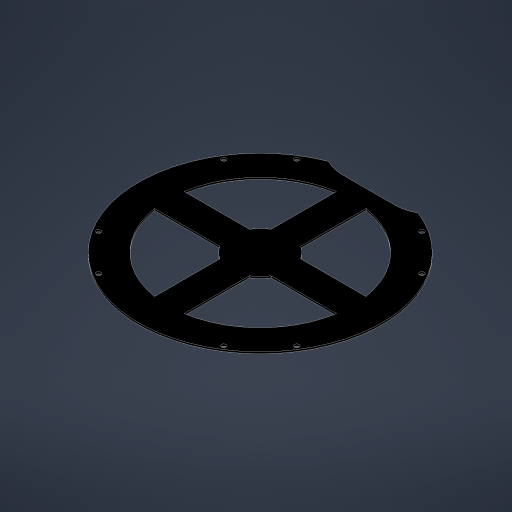
# Autodesk Inventor part: standart_sketch
Saved by Autodesk Inventor 2023 (Build 270158000, 158)
## iProperties
Created: 2022-10-10
Part Number: standart_sketch
Material: Generic
Document SubType Name: Modeling
Designer: braun
Density: 1 g/cm^3
Appearance: Default
Author: braun
Autodesk Inventor part; units mm, degrees
(part 1 of 2)
ref_plane "YZ Plane" through (0, 0, 0) normal (1, 0, 0) x (0, 1, 0)
ref_plane "XZ Plane" through (0, 0, 0) normal (0, 1, 0) x (-1, 0, 0)
ref_plane "XY Plane" through (0, 0, 0) normal (0, 0, 1) x (1, 0, 0)
sketch "Sketch2" plane through (0, 0, 0) normal (0, 1, 0) x (-1, 0, 0)
  circle A0 centre (0, 0) radius 110 construction
  arc A1 (43.0581, -98.5) -> (-43.0581, -98.5) centre (0, 0) ccw
  line L0 (0, -107.5) -> (0, -98.5) construction
  line L1 (0, -98.5) -> (0, -73.5) construction
  line L2 (0, -98.5) -> (-43.0581, -98.5) construction
  line L3 (0, -98.5) -> (43.0581, -98.5) construction
  line L4 (43.0581, -98.5) -> (-43.0581, -98.5) construction
  line L5 (-18.0581, -73.5) -> (18.0581, -73.5)
  arc A2 (43.0581, -98.5) -> (18.0581, -73.5) centre (18.0581, -98.5) ccw
  arc A3 (-18.0581, -73.5) -> (-43.0581, -98.5) centre (-18.0581, -98.5) ccw
  line L6 (0, 107.5) -> (0, 97.5) construction
  line L7 (0, 97.5) -> (-22.5, 97.5) construction
  line L8 (-22.5, 97.5) -> (-22.5, 82.5) construction
  line L9 (22.5, 82.5) -> (22.5, 97.5) construction
  line L10 (22.5, 90) -> (-22.5, 90) construction
  line L11 (15, 97.5) -> (-15, 97.5)
  line L12 (-15, 82.5) -> (15, 82.5)
  arc A4 (15, 82.5) -> (15, 97.5) centre (15, 90) ccw
  arc A5 (-15, 97.5) -> (-15, 82.5) centre (-15, 90) ccw
  line L13 (22.5, 82.5) -> (17.5, 82.5) construction
  line L14 (17.5, 82.5) -> (17.5, 77.5) construction
  circle A6 centre (17.5, 77.5) radius 1.6
  circle A7 centre (-17.5, 77.5) radius 1.6
  line L15 (-58.336309, 79.549513) -> (-79.549513, 58.336309)
  arc A8 (-47.729708, 68.942911) -> (-58.336309, 79.549513) centre (-53.033009, 74.246212) ccw
  arc A9 (-79.549513, 58.336309) -> (-68.942911, 47.729708) centre (-74.246212, 53.033009) ccw
  line L16 (-68.942911, 47.729708) -> (-47.729708, 68.942911)
  circle A10 centre (-67.175144, 42.426407) radius 1.6
  circle A11 centre (-42.426407, 67.175144) radius 1.6
  line L17 (-97.5, 15) -> (-97.5, -15)
  arc A12 (-82.5, 15) -> (-97.5, 15) centre (-90, 15) ccw
  arc A13 (-97.5, -15) -> (-82.5, -15) centre (-90, -15) ccw
  line L18 (-82.5, -15) -> (-82.5, 15)
  circle A14 centre (-77.5, -17.5) radius 1.6
  circle A15 centre (-77.5, 17.5) radius 1.6
  line L19 (-79.549513, -58.336309) -> (-58.336309, -79.549513)
  arc A16 (-68.942911, -47.729708) -> (-79.549513, -58.336309) centre (-74.246212, -53.033009) ccw
  arc A17 (-58.336309, -79.549513) -> (-47.729708, -68.942911) centre (-53.033009, -74.246212) ccw
  line L20 (-47.729708, -68.942911) -> (-68.942911, -47.729708)
  circle A18 centre (-42.426407, -67.175144) radius 1.6
  circle A19 centre (-67.175144, -42.426407) radius 1.6
  line L21 (-15, -97.5) -> (15, -97.5)
  arc A20 (-15, -82.5) -> (-15, -97.5) centre (-15, -90) ccw
  arc A21 (15, -97.5) -> (15, -82.5) centre (15, -90) ccw
  line L22 (15, -82.5) -> (-15, -82.5)
  circle A22 centre (17.5, -77.5) radius 1.6
  circle A23 centre (-17.5, -77.5) radius 1.6
  line L23 (58.336309, -79.549513) -> (79.549513, -58.336309)
  arc A24 (47.729708, -68.942911) -> (58.336309, -79.549513) centre (53.033009, -74.246212) ccw
  arc A25 (79.549513, -58.336309) -> (68.942911, -47.729708) centre (74.246212, -53.033009) ccw
  line L24 (68.942911, -47.729708) -> (47.729708, -68.942911)
  circle A26 centre (67.175144, -42.426407) radius 1.6
  circle A27 centre (42.426407, -67.175144) radius 1.6
  line L25 (97.5, -15) -> (97.5, 15)
  arc A28 (82.5, -15) -> (97.5, -15) centre (90, -15) ccw
  arc A29 (97.5, 15) -> (82.5, 15) centre (90, 15) ccw
  line L26 (82.5, 15) -> (82.5, -15)
  circle A30 centre (77.5, 17.5) radius 1.6
  circle A31 centre (77.5, -17.5) radius 1.6
  line L27 (79.549513, 58.336309) -> (58.336309, 79.549513)
  arc A32 (68.942911, 47.729708) -> (79.549513, 58.336309) centre (74.246212, 53.033009) ccw
  arc A33 (58.336309, 79.549513) -> (47.729708, 68.942911) centre (53.033009, 74.246212) ccw
  line L28 (47.729708, 68.942911) -> (68.942911, 47.729708)
  circle A34 centre (42.426407, 67.175144) radius 1.6
  circle A35 centre (67.175144, 42.426407) radius 1.6
  circle A36 centre (0, 0) radius 82.5
  line L29 (82.5, 0) -> (62.5, 0) construction
  line L30 (40.826407, 0) -> (40.826407, -10) construction
  line L31 (40.826407, 0) -> (40.826407, 10) construction
  line L32 (40.826407, -10) -> (17.320508, -10)
  line L33 (40.826407, -10) -> (61.694813, -10)
  line L34 (40.826407, 10) -> (17.320508, 10)
  line L35 (40.826407, 10) -> (61.694813, 10)
  line L36 (10, 40.826407) -> (10, 61.694813)
  line L37 (10, 40.826407) -> (10, 17.320508)
  line L38 (-10, 40.826407) -> (-10, 17.320508)
  line L39 (-10, 40.826407) -> (-10, 61.694813)
  line L40 (-40.826407, 10) -> (-61.694813, 10)
  line L41 (-40.826407, 10) -> (-17.320508, 10)
  line L42 (-40.826407, -10) -> (-17.320508, -10)
  line L43 (-40.826407, -10) -> (-61.694813, -10)
  line L44 (-10, -40.826407) -> (-10, -61.694813)
  line L45 (-10, -40.826407) -> (-10, -17.320508)
  line L46 (10, -40.826407) -> (10, -17.320508)
  line L47 (10, -40.826407) -> (10, -61.694813)
  arc A37 (10, -17.320508) -> (17.320508, -10) centre (0, 0) ccw
  arc A38 (-17.320508, -10) -> (-10, -17.320508) centre (0, 0) ccw
  arc A39 (17.320508, 10) -> (10, 17.320508) centre (0, 0) ccw
  arc A40 (-10, 17.320508) -> (-17.320508, 10) centre (0, 0) ccw
  arc A41 (61.694813, 10) -> (10, 61.694813) centre (0, 0) ccw
  arc A42 (-10, 61.694813) -> (-61.694813, 10) centre (0, 0) ccw
  arc A43 (-61.694813, -10) -> (-10, -61.694813) centre (0, 0) ccw
  arc A44 (10, -61.694813) -> (61.694813, -10) centre (0, 0) ccw
  point P0 (0, 90)
  point P1 (-45.961941, 70.710678)
  point P2 (-82.5, 17.5)
  point P3 (-70.710678, -45.961941)
  point P4 (-17.5, -82.5)
  point P5 (45.961941, -70.710678)
  point P6 (82.5, -17.5)
  point P7 (70.710678, 45.961941)
  point P8 (30.333369, -76.721162)
  point P9 (-30.333369, -76.721162)
  dimension "d34" = 220
  dimension "d35" = 215
  dimension "d36" = 9
  dimension "d37" = 25
  dimension "d38" = 10
  dimension "d39" = 22.5
  dimension "d40" = 15
  dimension "d41" = 45
  dimension "d42" = 5
  dimension "d43" = 5
  dimension "d44" = 3.2
  dimension "d45" = 86.1162
  dimension "d46" = 45
  dimension "d47" = 360
  dimension "d48" = 20
  dimension "d50" = 10
  dimension "d51" = 10
  dimension "d54" = 360
  constraints: 100 end point, 59 point on circle, 44 centre point, 18 point on line, 6 coincident, 6 tangent, 5 midpoint, 5 vertical, 4 horizontal, 2 parallel, 1 collinear, 1 perpendicular, 1 symmetric about line, 166 other
  measures "d34" diameter of A0
  measures "d35" diameter of A1
  measures "d36" distance of L0.start L0.end
  measures "d37" distance of L0.end L1.end
  measures "d38" distance of L6.start L6.end
  measures "d39" distance of L6.end L7.end
  measures "d40" distance of L7.end L8.end
  measures "d41" distance of L8.end L9.start
  measures "d42" distance of L9.start L13.end
  measures "d43" distance of L13.end L14.end
  measures "d44" diameter of A6
  measures "d45" distance of L3.end L2.end
  measures "d46" distance of L10.start L10.end
  measures "d48" distance of L29.start L29.end
  measures "d50" distance of L30.start L30.end
  measures "d51" distance of L30.start L31.end
extrude "Extrusion2" add sketch "Sketch2" along normal blind 1.2 contours A2 L5 A3 A36 | A6 | A7 | A14 | A15 | A30 | A31 picked at (-5.106963, 5.928675)
sketch "Sketch3" plane through (0, 1.2, 0) normal (0, 1, 0) x (1, 0, 0)
  arc A0 (-30.333369, 76.721162) -> (30.333369, 76.721162) centre (0, 0) ccw construction
  line L0 (0, -79.5) -> (2.5, -79.5)
  line L1 (2.5, -79.5) -> (2.5, -70.8)
  line L2 (2.5, -70.8) -> (-2.5, -70.8)
  line L3 (-2.5, -70.8) -> (-2.5, -79.5)
  line L4 (-2.5, -79.5) -> (0, -79.5)
  line L5 (5.5, -73.75) -> (6.4, -73.75)
  line L6 (6.4, -73.75) -> (6.4, -76.55)
  line L7 (6.4, -76.55) -> (4.6, -76.55)
  line L8 (4.6, -76.55) -> (4.6, -73.75)
  line L9 (4.6, -73.75) -> (5.5, -73.75)
  line L10 (-5.5, -73.75) -> (-6.4, -73.75)
  line L11 (-6.4, -73.75) -> (-6.4, -76.55)
  line L12 (-6.4, -76.55) -> (-4.6, -76.55)
  line L13 (-4.6, -76.55) -> (-4.6, -73.75)
  line L14 (-4.6, -73.75) -> (-5.5, -73.75)
  line L15 (-5.5, -71.15) -> (-3.25, -71.15)
  line L16 (-3.25, -71.15) -> (-3.25, -69.55)
  line L17 (-3.25, -69.55) -> (-7.75, -69.55)
  line L18 (-7.75, -69.55) -> (-7.75, -71.15)
  line L19 (-7.75, -71.15) -> (-5.5, -71.15)
  line L20 (5.5, -71.15) -> (3.25, -71.15)
  line L21 (3.25, -71.15) -> (3.25, -69.55)
  line L22 (3.25, -69.55) -> (7.75, -69.55)
  line L23 (7.75, -69.55) -> (7.75, -71.15)
  line L24 (7.75, -71.15) -> (5.5, -71.15)
  line L25 (-5.5, -79.15) -> (-3.25, -79.15)
  line L26 (-3.25, -79.15) -> (-3.25, -80.75)
  line L27 (-3.25, -80.75) -> (-7.75, -80.75)
  line L28 (-7.75, -80.75) -> (-7.75, -79.15)
  line L29 (-7.75, -79.15) -> (-5.5, -79.15)
  line L30 (27.286785, -74.368786) -> (27.899079, -75.846993)
  line L31 (25.208056, -75.229824) -> (27.286785, -74.368786)
  line L32 (23.381588, -73.172152) -> (25.044571, -72.483322)
  line L33 (25.044571, -72.483322) -> (23.973057, -69.896459)
  line L34 (23.129327, -76.090862) -> (25.208056, -75.229824)
  line L35 (27.899079, -75.846993) -> (23.741621, -77.569069)
  line L36 (23.741621, -77.569069) -> (23.129327, -76.090862)
  line L37 (23.973057, -69.896459) -> (23.141566, -70.240874)
  line L38 (22.310074, -70.585289) -> (23.381588, -73.172152)
  line L39 (24.784288, -66.367379) -> (28.113634, -74.405131)
  line L40 (22.146589, -67.838788) -> (24.225318, -66.97775)
  line L41 (32.733032, -72.491714) -> (29.403686, -64.453962)
  line L42 (29.403686, -64.453962) -> (24.784288, -66.367379)
  line L43 (23.141566, -70.240874) -> (22.310074, -70.585289)
  line L44 (28.113634, -74.405131) -> (30.423333, -73.448423)
  line L45 (20.06786, -68.699825) -> (22.146589, -67.838788)
  line L46 (24.225318, -66.97775) -> (23.613024, -65.499543)
  line L47 (23.613024, -65.499543) -> (19.455566, -67.221618)
  line L48 (19.455566, -67.221618) -> (20.06786, -68.699825)
  line L49 (33.304241, -66.031357) -> (34.135732, -65.686942)
  line L50 (34.135732, -65.686942) -> (35.207246, -68.273804)
  line L51 (35.207246, -68.273804) -> (33.544263, -68.962634)
  line L52 (33.544263, -68.962634) -> (32.472749, -66.375772)
  line L53 (32.472749, -66.375772) -> (33.304241, -66.031357)
  line L54 (30.230535, -64.490308) -> (29.618241, -63.0121)
  line L55 (32.309264, -63.62927) -> (30.230535, -64.490308)
  line L56 (34.387993, -62.768232) -> (32.309264, -63.62927)
  line L57 (33.775699, -61.290025) -> (34.387993, -62.768232)
  line L58 (29.618241, -63.0121) -> (33.775699, -61.290025)
  line L59 (30.423333, -73.448423) -> (32.733032, -72.491714)
  line L60 (53.669405, -58.265599) -> (54.800776, -59.39697)
  line L61 (52.078414, -59.856589) -> (53.669405, -58.265599)
  line L62 (49.603541, -58.654507) -> (50.876333, -57.381715)
  line L63 (50.876333, -57.381715) -> (48.896434, -55.401816)
  line L64 (50.487424, -61.447579) -> (52.078414, -59.856589)
  line L65 (54.800776, -59.39697) -> (51.618795, -62.57895)
  line L66 (51.618795, -62.57895) -> (50.487424, -61.447579)
  line L67 (48.896434, -55.401816) -> (48.260038, -56.038212)
  line L68 (47.623642, -56.674609) -> (49.603541, -58.654507)
  line L69 (48.295393, -51.830927) -> (54.447222, -57.982756)
  line L70 (46.42156, -54.199735) -> (48.01255, -52.608745)
  line L71 (57.982756, -54.447222) -> (51.830927, -48.295393)
  line L72 (51.830927, -48.295393) -> (48.295393, -51.830927)
  line L73 (48.260038, -56.038212) -> (47.623642, -56.674609)
  line L74 (54.447222, -57.982756) -> (56.214989, -56.214989)
  line L75 (44.83057, -55.790725) -> (46.42156, -54.199735)
  line L76 (48.01255, -52.608745) -> (46.88118, -51.477374)
  line L77 (46.88118, -51.477374) -> (43.699199, -54.659354)
  line L78 (43.699199, -54.659354) -> (44.83057, -55.790725)
  line L79 (56.038212, -48.260038) -> (56.674609, -47.623642)
  line L80 (56.674609, -47.623642) -> (58.654507, -49.603541)
  line L81 (58.654507, -49.603541) -> (57.381715, -50.876333)
  line L82 (57.381715, -50.876333) -> (55.401816, -48.896434)
  line L83 (55.401816, -48.896434) -> (56.038212, -48.260038)
  line L84 (52.608745, -48.01255) -> (51.477374, -46.88118)
  line L85 (54.199735, -46.42156) -> (52.608745, -48.01255)
  line L86 (55.790725, -44.83057) -> (54.199735, -46.42156)
  line L87 (54.659354, -43.699199) -> (55.790725, -44.83057)
  line L88 (51.477374, -46.88118) -> (54.659354, -43.699199)
  line L89 (56.214989, -56.214989) -> (57.982756, -54.447222)
  line L90 (71.881344, -33.292002) -> (73.359551, -33.904296)
  line L91 (71.020306, -35.370731) -> (71.881344, -33.292002)
  line L92 (68.273804, -35.207246) -> (68.962634, -33.544263)
  line L93 (68.962634, -33.544263) -> (66.375772, -32.472749)
  line L94 (70.159268, -37.44946) -> (71.020306, -35.370731)
  line L95 (73.359551, -33.904296) -> (71.637476, -38.061754)
  line L96 (71.637476, -38.061754) -> (70.159268, -37.44946)
  line L97 (66.375772, -32.472749) -> (66.031357, -33.304241)
  line L98 (65.686942, -34.135732) -> (68.273804, -35.207246)
  line L99 (64.453962, -29.403686) -> (72.491714, -32.733032)
  line L100 (63.62927, -32.309264) -> (64.490308, -30.230535)
  line L101 (74.405131, -28.113634) -> (66.367379, -24.784288)
  line L102 (66.367379, -24.784288) -> (64.453962, -29.403686)
  line L103 (66.031357, -33.304241) -> (65.686942, -34.135732)
  line L104 (72.491714, -32.733032) -> (73.448423, -30.423333)
  line L105 (62.768232, -34.387993) -> (63.62927, -32.309264)
  line L106 (64.490308, -30.230535) -> (63.0121, -29.618241)
  line L107 (63.0121, -29.618241) -> (61.290025, -33.775699)
  line L108 (61.290025, -33.775699) -> (62.768232, -34.387993)
  line L109 (70.240874, -23.141566) -> (70.585289, -22.310074)
  line L110 (70.585289, -22.310074) -> (73.172152, -23.381588)
  line L111 (73.172152, -23.381588) -> (72.483322, -25.044571)
  line L112 (72.483322, -25.044571) -> (69.896459, -23.973057)
  line L113 (69.896459, -23.973057) -> (70.240874, -23.141566)
  line L114 (66.97775, -24.225318) -> (65.499543, -23.613024)
  line L115 (67.838788, -22.146589) -> (66.97775, -24.225318)
  line L116 (68.699825, -20.06786) -> (67.838788, -22.146589)
  line L117 (67.221618, -19.455566) -> (68.699825, -20.06786)
  line L118 (65.499543, -23.613024) -> (67.221618, -19.455566)
  line L119 (73.448423, -30.423333) -> (74.405131, -28.113634)
  arc A1 (-30.333369, 76.721162) -> (-18.0581, 73.5) centre (-18.0581, 98.5) ccw
  line L120 (18.0581, 73.5) -> (-18.0581, 73.5) construction
  line L121 (0, 0) -> (0, -9) construction
  line L122 (0, -79.5) -> (0, -82.5) construction
  line L123 (0, 73.5) -> (0, 70.5) construction
  line L124 (0, 70.5) -> (2.5, 70.5)
  line L125 (2.5, 70.5) -> (2.5, 61.8)
  line L126 (2.5, 61.8) -> (-2.5, 61.8)
  line L127 (-2.5, 61.8) -> (-2.5, 70.5)
  line L128 (-2.5, 70.5) -> (0, 70.5)
  line L129 (5.5, 66.15) -> (5.5, 70.95) construction
  line L130 (5.5, 66.15) -> (5.5, 61.35) construction
  line L131 (0, -75.15) -> (0, -64.15) construction
  line L132 (0, -64.15) -> (3.25, -64.15) construction
  line L133 (0, -48.8) -> (2.5, -48.8)
  line L134 (2.5, -48.8) -> (2.5, -57.5)
  line L135 (2.5, -57.5) -> (-2.5, -57.5)
  line L136 (-2.5, -57.5) -> (-2.5, -48.8)
  line L137 (-2.5, -48.8) -> (0, -48.8)
  line L138 (5.5, -54.55) -> (6.4, -54.55)
  line L139 (6.4, -54.55) -> (6.4, -51.75)
  line L140 (6.4, -51.75) -> (4.6, -51.75)
  line L141 (4.6, -51.75) -> (4.6, -54.55)
  line L142 (4.6, -54.55) -> (5.5, -54.55)
  line L143 (-4.6, -54.55) -> (-5.5, -54.55)
  line L144 (-5.5, -54.55) -> (-6.4, -54.55)
  line L145 (-4.6, -51.75) -> (-4.6, -54.55)
  line L146 (-6.4, -51.75) -> (-4.6, -51.75)
  line L147 (-6.4, -54.55) -> (-6.4, -51.75)
  line L148 (-5.5, -57.15) -> (-3.25, -57.15)
  line L149 (-3.25, -57.15) -> (-3.25, -58.75)
  line L150 (-3.25, -58.75) -> (-7.75, -58.75)
  line L151 (-7.75, -58.75) -> (-7.75, -57.15)
  line L152 (-7.75, -57.15) -> (-5.5, -57.15)
  line L153 (5.5, -57.15) -> (3.25, -57.15)
  line L154 (3.25, -57.15) -> (3.25, -58.75)
  line L155 (7.75, -57.15) -> (5.5, -57.15)
  line L156 (3.25, -58.75) -> (7.75, -58.75)
  line L157 (7.75, -58.75) -> (7.75, -57.15)
  line L158 (-3.25, -47.55) -> (-7.75, -47.55)
  line L159 (-5.5, -49.15) -> (-3.25, -49.15)
  line L160 (-7.75, -49.15) -> (-5.5, -49.15)
  line L161 (-7.75, -47.55) -> (-7.75, -49.15)
  line L162 (-3.25, -49.15) -> (-3.25, -47.55)
  line L163 (23.741621, -50.730931) -> (23.129327, -52.209138)
  line L164 (23.973057, -58.403541) -> (23.141566, -58.059126)
  line L165 (22.310074, -57.714711) -> (23.381588, -55.127848)
  line L166 (22.146589, -60.461212) -> (24.225318, -61.32225)
  line L167 (23.141566, -58.059126) -> (22.310074, -57.714711)
  line L168 (20.06786, -59.600175) -> (22.146589, -60.461212)
  line L169 (24.225318, -61.32225) -> (23.613024, -62.800457)
  line L170 (23.613024, -62.800457) -> (19.455566, -61.078382)
  line L171 (19.455566, -61.078382) -> (20.06786, -59.600175)
  line L172 (0, -48.8) -> (0, -45.8) construction
  line L173 (0, -53.15) -> (0, -64.15) construction
  line L174 (79.15, -3.25) -> (80.75, -3.25)
  line L175 (79.15, -5.5) -> (79.15, -3.25)
  line L176 (76.55, -6.4) -> (76.55, -4.6)
  line L177 (76.55, -4.6) -> (73.75, -4.6)
  line L178 (79.15, -7.75) -> (79.15, -5.5)
  line L179 (80.75, -3.25) -> (80.75, -7.75)
  line L180 (80.75, -7.75) -> (79.15, -7.75)
  line L181 (73.75, -4.6) -> (73.75, -5.5)
  line L182 (73.75, -6.4) -> (76.55, -6.4)
  line L183 (70.8, -2.5) -> (79.5, -2.5)
  line L184 (71.15, -5.5) -> (71.15, -3.25)
  line L185 (79.5, 2.5) -> (70.8, 2.5)
  line L186 (70.8, 2.5) -> (70.8, -2.5)
  line L187 (73.75, -5.5) -> (73.75, -6.4)
  line L188 (79.5, -2.5) -> (79.5, 0)
  line L189 (71.15, -7.75) -> (71.15, -5.5)
  line L190 (71.15, -3.25) -> (69.55, -3.25)
  line L191 (69.55, -3.25) -> (69.55, -7.75)
  line L192 (69.55, -7.75) -> (71.15, -7.75)
  line L193 (73.75, 5.5) -> (73.75, 6.4)
  line L194 (73.75, 6.4) -> (76.55, 6.4)
  line L195 (76.55, 6.4) -> (76.55, 4.6)
  line L196 (76.55, 4.6) -> (73.75, 4.6)
  line L197 (73.75, 4.6) -> (73.75, 5.5)
  line L198 (71.15, 3.25) -> (69.55, 3.25)
  line L199 (71.15, 5.5) -> (71.15, 3.25)
  line L200 (71.15, 7.75) -> (71.15, 5.5)
  line L201 (69.55, 7.75) -> (71.15, 7.75)
  line L202 (69.55, 3.25) -> (69.55, 7.75)
  line L203 (79.5, 0) -> (79.5, 2.5)
  line L204 (74.368786, 27.286785) -> (75.846993, 27.899079)
  line L205 (75.229824, 25.208056) -> (74.368786, 27.286785)
  line L206 (73.172152, 23.381588) -> (72.483322, 25.044571)
  line L207 (72.483322, 25.044571) -> (69.896459, 23.973057)
  line L208 (76.090862, 23.129327) -> (75.229824, 25.208056)
  line L209 (75.846993, 27.899079) -> (77.569069, 23.741621)
  line L210 (77.569069, 23.741621) -> (76.090862, 23.129327)
  line L211 (69.896459, 23.973057) -> (70.240874, 23.141566)
  line L212 (70.585289, 22.310074) -> (73.172152, 23.381588)
  line L213 (66.367379, 24.784288) -> (74.405131, 28.113634)
  line L214 (67.838788, 22.146589) -> (66.97775, 24.225318)
  line L215 (72.491714, 32.733032) -> (64.453962, 29.403686)
  line L216 (64.453962, 29.403686) -> (66.367379, 24.784288)
  line L217 (70.240874, 23.141566) -> (70.585289, 22.310074)
  line L218 (74.405131, 28.113634) -> (73.448423, 30.423333)
  line L219 (68.699825, 20.06786) -> (67.838788, 22.146589)
  line L220 (66.97775, 24.225318) -> (65.499543, 23.613024)
  line L221 (65.499543, 23.613024) -> (67.221618, 19.455566)
  line L222 (67.221618, 19.455566) -> (68.699825, 20.06786)
  line L223 (66.031357, 33.304241) -> (65.686942, 34.135732)
  line L224 (65.686942, 34.135732) -> (68.273804, 35.207246)
  line L225 (68.273804, 35.207246) -> (68.962634, 33.544263)
  line L226 (68.962634, 33.544263) -> (66.375772, 32.472749)
  line L227 (66.375772, 32.472749) -> (66.031357, 33.304241)
  line L228 (64.490308, 30.230535) -> (63.0121, 29.618241)
  line L229 (63.62927, 32.309264) -> (64.490308, 30.230535)
  line L230 (62.768232, 34.387993) -> (63.62927, 32.309264)
  line L231 (61.290025, 33.775699) -> (62.768232, 34.387993)
  line L232 (63.0121, 29.618241) -> (61.290025, 33.775699)
  line L233 (73.448423, 30.423333) -> (72.491714, 32.733032)
  line L234 (58.265599, 53.669405) -> (59.39697, 54.800776)
  line L235 (59.856589, 52.078414) -> (58.265599, 53.669405)
  line L236 (58.654507, 49.603541) -> (57.381715, 50.876333)
  line L237 (57.381715, 50.876333) -> (55.401816, 48.896434)
  line L238 (61.447579, 50.487424) -> (59.856589, 52.078414)
  line L239 (59.39697, 54.800776) -> (62.57895, 51.618795)
  line L240 (62.57895, 51.618795) -> (61.447579, 50.487424)
  line L241 (55.401816, 48.896434) -> (56.038212, 48.260038)
  line L242 (56.674609, 47.623642) -> (58.654507, 49.603541)
  line L243 (51.830927, 48.295393) -> (57.982756, 54.447222)
  line L244 (54.199735, 46.42156) -> (52.608745, 48.01255)
  line L245 (54.447222, 57.982756) -> (48.295393, 51.830927)
  line L246 (48.295393, 51.830927) -> (51.830927, 48.295393)
  line L247 (56.038212, 48.260038) -> (56.674609, 47.623642)
  line L248 (57.982756, 54.447222) -> (56.214989, 56.214989)
  line L249 (55.790725, 44.83057) -> (54.199735, 46.42156)
  line L250 (52.608745, 48.01255) -> (51.477374, 46.88118)
  line L251 (51.477374, 46.88118) -> (54.659354, 43.699199)
  line L252 (54.659354, 43.699199) -> (55.790725, 44.83057)
  line L253 (48.260038, 56.038212) -> (47.623642, 56.674609)
  line L254 (47.623642, 56.674609) -> (49.603541, 58.654507)
  line L255 (49.603541, 58.654507) -> (50.876333, 57.381715)
  line L256 (50.876333, 57.381715) -> (48.896434, 55.401816)
  line L257 (48.896434, 55.401816) -> (48.260038, 56.038212)
  line L258 (48.01255, 52.608745) -> (46.88118, 51.477374)
  line L259 (46.42156, 54.199735) -> (48.01255, 52.608745)
  line L260 (44.83057, 55.790725) -> (46.42156, 54.199735)
  line L261 (43.699199, 54.659354) -> (44.83057, 55.790725)
  line L262 (46.88118, 51.477374) -> (43.699199, 54.659354)
  line L263 (56.214989, 56.214989) -> (54.447222, 57.982756)
  line L264 (33.292002, 71.881344) -> (33.904296, 73.359551)
  line L265 (35.370731, 71.020306) -> (33.292002, 71.881344)
  line L266 (35.207246, 68.273804) -> (33.544263, 68.962634)
  line L267 (33.544263, 68.962634) -> (32.472749, 66.375772)
  line L268 (37.44946, 70.159268) -> (35.370731, 71.020306)
  line L269 (33.904296, 73.359551) -> (38.061754, 71.637476)
  line L270 (38.061754, 71.637476) -> (37.44946, 70.159268)
  line L271 (32.472749, 66.375772) -> (33.304241, 66.031357)
  line L272 (34.135732, 65.686942) -> (35.207246, 68.273804)
  line L273 (29.403686, 64.453962) -> (32.733032, 72.491714)
  line L274 (32.309264, 63.62927) -> (30.230535, 64.490308)
  line L275 (28.113634, 74.405131) -> (24.784288, 66.367379)
  line L276 (24.784288, 66.367379) -> (29.403686, 64.453962)
  line L277 (33.304241, 66.031357) -> (34.135732, 65.686942)
  line L278 (32.733032, 72.491714) -> (30.423333, 73.448423)
  line L279 (34.387993, 62.768232) -> (32.309264, 63.62927)
  line L280 (30.230535, 64.490308) -> (29.618241, 63.0121)
  line L281 (29.618241, 63.0121) -> (33.775699, 61.290025)
  line L282 (33.775699, 61.290025) -> (34.387993, 62.768232)
  line L283 (23.141566, 70.240874) -> (22.310074, 70.585289)
  line L284 (22.310074, 70.585289) -> (23.381588, 73.172152)
  line L285 (23.381588, 73.172152) -> (25.044571, 72.483322)
  line L286 (25.044571, 72.483322) -> (23.973057, 69.896459)
  line L287 (23.973057, 69.896459) -> (23.141566, 70.240874)
  line L288 (24.225318, 66.97775) -> (23.613024, 65.499543)
  line L289 (22.146589, 67.838788) -> (24.225318, 66.97775)
  line L290 (20.06786, 68.699825) -> (22.146589, 67.838788)
  line L291 (19.455566, 67.221618) -> (20.06786, 68.699825)
  line L292 (23.613024, 65.499543) -> (19.455566, 67.221618)
  line L293 (30.423333, 73.448423) -> (28.113634, 74.405131)
  line L294 (3.25, 79.15) -> (3.25, 80.75)
  line L295 (5.5, 79.15) -> (3.25, 79.15)
  line L296 (6.4, 76.55) -> (4.6, 76.55)
  line L297 (4.6, 76.55) -> (4.6, 73.75)
  line L298 (7.75, 79.15) -> (5.5, 79.15)
  line L299 (3.25, 80.75) -> (7.75, 80.75)
  line L300 (7.75, 80.75) -> (7.75, 79.15)
  line L301 (4.6, 73.75) -> (5.5, 73.75)
  line L302 (6.4, 73.75) -> (6.4, 76.55)
  line L303 (2.5, 70.8) -> (2.5, 79.5)
  line L304 (5.5, 71.15) -> (3.25, 71.15)
  line L305 (-2.5, 79.5) -> (-2.5, 70.8)
  line L306 (-2.5, 70.8) -> (2.5, 70.8)
  line L307 (5.5, 73.75) -> (6.4, 73.75)
  line L308 (2.5, 79.5) -> (0, 79.5)
  line L309 (7.75, 71.15) -> (5.5, 71.15)
  line L310 (3.25, 71.15) -> (3.25, 69.55)
  line L311 (3.25, 69.55) -> (7.75, 69.55)
  line L312 (7.75, 69.55) -> (7.75, 71.15)
  line L313 (-5.5, 73.75) -> (-6.4, 73.75)
  line L314 (-6.4, 73.75) -> (-6.4, 76.55)
  line L315 (-6.4, 76.55) -> (-4.6, 76.55)
  line L316 (-4.6, 76.55) -> (-4.6, 73.75)
  line L317 (-4.6, 73.75) -> (-5.5, 73.75)
  line L318 (-3.25, 71.15) -> (-3.25, 69.55)
  line L319 (-5.5, 71.15) -> (-3.25, 71.15)
  line L320 (-7.75, 71.15) -> (-5.5, 71.15)
  line L321 (-7.75, 69.55) -> (-7.75, 71.15)
  line L322 (-3.25, 69.55) -> (-7.75, 69.55)
  line L323 (0, 79.5) -> (-2.5, 79.5)
  line L324 (-27.286785, 74.368786) -> (-27.899079, 75.846993)
  line L325 (-25.208056, 75.229824) -> (-27.286785, 74.368786)
  line L326 (-23.381588, 73.172152) -> (-25.044571, 72.483322)
  line L327 (-25.044571, 72.483322) -> (-23.973057, 69.896459)
  line L328 (-23.129327, 76.090862) -> (-25.208056, 75.229824)
  line L329 (-27.899079, 75.846993) -> (-23.741621, 77.569069)
  line L330 (-23.741621, 77.569069) -> (-23.129327, 76.090862)
  line L331 (-23.973057, 69.896459) -> (-23.141566, 70.240874)
  line L332 (-22.310074, 70.585289) -> (-23.381588, 73.172152)
  line L333 (-24.784288, 66.367379) -> (-28.113634, 74.405131)
  line L334 (-22.146589, 67.838788) -> (-24.225318, 66.97775)
  line L335 (-32.733032, 72.491714) -> (-29.403686, 64.453962)
  line L336 (-29.403686, 64.453962) -> (-24.784288, 66.367379)
  line L337 (-23.141566, 70.240874) -> (-22.310074, 70.585289)
  line L338 (-28.113634, 74.405131) -> (-30.423333, 73.448423)
  line L339 (-20.06786, 68.699825) -> (-22.146589, 67.838788)
  line L340 (-24.225318, 66.97775) -> (-23.613024, 65.499543)
  line L341 (-23.613024, 65.499543) -> (-19.455566, 67.221618)
  line L342 (-19.455566, 67.221618) -> (-20.06786, 68.699825)
  line L343 (-33.304241, 66.031357) -> (-34.135732, 65.686942)
  line L344 (-34.135732, 65.686942) -> (-35.207246, 68.273804)
  line L345 (-35.207246, 68.273804) -> (-33.544263, 68.962634)
  line L346 (-33.544263, 68.962634) -> (-32.472749, 66.375772)
  line L347 (-32.472749, 66.375772) -> (-33.304241, 66.031357)
  line L348 (-30.230535, 64.490308) -> (-29.618241, 63.0121)
  line L349 (-32.309264, 63.62927) -> (-30.230535, 64.490308)
  line L350 (-34.387993, 62.768232) -> (-32.309264, 63.62927)
  line L351 (-33.775699, 61.290025) -> (-34.387993, 62.768232)
  line L352 (-29.618241, 63.0121) -> (-33.775699, 61.290025)
  line L353 (-30.423333, 73.448423) -> (-32.733032, 72.491714)
  line L354 (-53.669405, 58.265599) -> (-54.800776, 59.39697)
  line L355 (-52.078414, 59.856589) -> (-53.669405, 58.265599)
  line L356 (-49.603541, 58.654507) -> (-50.876333, 57.381715)
  line L357 (-50.876333, 57.381715) -> (-48.896434, 55.401816)
  line L358 (-50.487424, 61.447579) -> (-52.078414, 59.856589)
  line L359 (-54.800776, 59.39697) -> (-51.618795, 62.57895)
  line L360 (-51.618795, 62.57895) -> (-50.487424, 61.447579)
  line L361 (-48.896434, 55.401816) -> (-48.260038, 56.038212)
  line L362 (-47.623642, 56.674609) -> (-49.603541, 58.654507)
  line L363 (-48.295393, 51.830927) -> (-54.447222, 57.982756)
  line L364 (-46.42156, 54.199735) -> (-48.01255, 52.608745)
  line L365 (-57.982756, 54.447222) -> (-51.830927, 48.295393)
  line L366 (-51.830927, 48.295393) -> (-48.295393, 51.830927)
  line L367 (-48.260038, 56.038212) -> (-47.623642, 56.674609)
  line L368 (-54.447222, 57.982756) -> (-56.214989, 56.214989)
  line L369 (-44.83057, 55.790725) -> (-46.42156, 54.199735)
  line L370 (-48.01255, 52.608745) -> (-46.88118, 51.477374)
  line L371 (-46.88118, 51.477374) -> (-43.699199, 54.659354)
  line L372 (-43.699199, 54.659354) -> (-44.83057, 55.790725)
  line L373 (-56.038212, 48.260038) -> (-56.674609, 47.623642)
  line L374 (-56.674609, 47.623642) -> (-58.654507, 49.603541)
  line L375 (-58.654507, 49.603541) -> (-57.381715, 50.876333)
  line L376 (-57.381715, 50.876333) -> (-55.401816, 48.896434)
  line L377 (-55.401816, 48.896434) -> (-56.038212, 48.260038)
  line L378 (-52.608745, 48.01255) -> (-51.477374, 46.88118)
  line L379 (-54.199735, 46.42156) -> (-52.608745, 48.01255)
  line L380 (-55.790725, 44.83057) -> (-54.199735, 46.42156)
  line L381 (-54.659354, 43.699199) -> (-55.790725, 44.83057)
  line L382 (-51.477374, 46.88118) -> (-54.659354, 43.699199)
  line L383 (-56.214989, 56.214989) -> (-57.982756, 54.447222)
  line L384 (-71.881344, 33.292002) -> (-73.359551, 33.904296)
  line L385 (-71.020306, 35.370731) -> (-71.881344, 33.292002)
  line L386 (-68.273804, 35.207246) -> (-68.962634, 33.544263)
  line L387 (-68.962634, 33.544263) -> (-66.375772, 32.472749)
  line L388 (-70.159268, 37.44946) -> (-71.020306, 35.370731)
  line L389 (-73.359551, 33.904296) -> (-71.637476, 38.061754)
  line L390 (-71.637476, 38.061754) -> (-70.159268, 37.44946)
  line L391 (-66.375772, 32.472749) -> (-66.031357, 33.304241)
  line L392 (-65.686942, 34.135732) -> (-68.273804, 35.207246)
  line L393 (-64.453962, 29.403686) -> (-72.491714, 32.733032)
  line L394 (-63.62927, 32.309264) -> (-64.490308, 30.230535)
  line L395 (-74.405131, 28.113634) -> (-66.367379, 24.784288)
  line L396 (-66.367379, 24.784288) -> (-64.453962, 29.403686)
  line L397 (-66.031357, 33.304241) -> (-65.686942, 34.135732)
  line L398 (-72.491714, 32.733032) -> (-73.448423, 30.423333)
  line L399 (-62.768232, 34.387993) -> (-63.62927, 32.309264)
  line L400 (-64.490308, 30.230535) -> (-63.0121, 29.618241)
  line L401 (-63.0121, 29.618241) -> (-61.290025, 33.775699)
  line L402 (-61.290025, 33.775699) -> (-62.768232, 34.387993)
  line L403 (-70.240874, 23.141566) -> (-70.585289, 22.310074)
  line L404 (-70.585289, 22.310074) -> (-73.172152, 23.381588)
  line L405 (-73.172152, 23.381588) -> (-72.483322, 25.044571)
  line L406 (-72.483322, 25.044571) -> (-69.896459, 23.973057)
  line L407 (-69.896459, 23.973057) -> (-70.240874, 23.141566)
  line L408 (-66.97775, 24.225318) -> (-65.499543, 23.613024)
  line L409 (-67.838788, 22.146589) -> (-66.97775, 24.225318)
  line L410 (-68.699825, 20.06786) -> (-67.838788, 22.146589)
  line L411 (-67.221618, 19.455566) -> (-68.699825, 20.06786)
  line L412 (-65.499543, 23.613024) -> (-67.221618, 19.455566)
  line L413 (-73.448423, 30.423333) -> (-74.405131, 28.113634)
  line L414 (-79.15, 3.25) -> (-80.75, 3.25)
  line L415 (-79.15, 5.5) -> (-79.15, 3.25)
  line L416 (-76.55, 6.4) -> (-76.55, 4.6)
  line L417 (-76.55, 4.6) -> (-73.75, 4.6)
  line L418 (-79.15, 7.75) -> (-79.15, 5.5)
  line L419 (-80.75, 3.25) -> (-80.75, 7.75)
  line L420 (-80.75, 7.75) -> (-79.15, 7.75)
  line L421 (-73.75, 4.6) -> (-73.75, 5.5)
  line L422 (-73.75, 6.4) -> (-76.55, 6.4)
  line L423 (-70.8, 2.5) -> (-79.5, 2.5)
  line L424 (-71.15, 5.5) -> (-71.15, 3.25)
  line L425 (-79.5, -2.5) -> (-70.8, -2.5)
  line L426 (-70.8, -2.5) -> (-70.8, 2.5)
  line L427 (-73.75, 5.5) -> (-73.75, 6.4)
  line L428 (-79.5, 2.5) -> (-79.5, 0)
  line L429 (-71.15, 7.75) -> (-71.15, 5.5)
  line L430 (-71.15, 3.25) -> (-69.55, 3.25)
  line L431 (-69.55, 3.25) -> (-69.55, 7.75)
  line L432 (-69.55, 7.75) -> (-71.15, 7.75)
  line L433 (-73.75, -5.5) -> (-73.75, -6.4)
  line L434 (-73.75, -6.4) -> (-76.55, -6.4)
  line L435 (-76.55, -6.4) -> (-76.55, -4.6)
  line L436 (-76.55, -4.6) -> (-73.75, -4.6)
  line L437 (-73.75, -4.6) -> (-73.75, -5.5)
  line L438 (-71.15, -3.25) -> (-69.55, -3.25)
  line L439 (-71.15, -5.5) -> (-71.15, -3.25)
  line L440 (-71.15, -7.75) -> (-71.15, -5.5)
  line L441 (-69.55, -7.75) -> (-71.15, -7.75)
  line L442 (-69.55, -3.25) -> (-69.55, -7.75)
  line L443 (-79.5, 0) -> (-79.5, -2.5)
  line L444 (-74.368786, -27.286785) -> (-75.846993, -27.899079)
  line L445 (-75.229824, -25.208056) -> (-74.368786, -27.286785)
  line L446 (-73.172152, -23.381588) -> (-72.483322, -25.044571)
  line L447 (-72.483322, -25.044571) -> (-69.896459, -23.973057)
  line L448 (-76.090862, -23.129327) -> (-75.229824, -25.208056)
  line L449 (-75.846993, -27.899079) -> (-77.569069, -23.741621)
  line L450 (-77.569069, -23.741621) -> (-76.090862, -23.129327)
  line L451 (-69.896459, -23.973057) -> (-70.240874, -23.141566)
  line L452 (-70.585289, -22.310074) -> (-73.172152, -23.381588)
  line L453 (-66.367379, -24.784288) -> (-74.405131, -28.113634)
  line L454 (-67.838788, -22.146589) -> (-66.97775, -24.225318)
  line L455 (-72.491714, -32.733032) -> (-64.453962, -29.403686)
  line L456 (-64.453962, -29.403686) -> (-66.367379, -24.784288)
  line L457 (-70.240874, -23.141566) -> (-70.585289, -22.310074)
  line L458 (-74.405131, -28.113634) -> (-73.448423, -30.423333)
  line L459 (-68.699825, -20.06786) -> (-67.838788, -22.146589)
  line L460 (-66.97775, -24.225318) -> (-65.499543, -23.613024)
  line L461 (-65.499543, -23.613024) -> (-67.221618, -19.455566)
  line L462 (-67.221618, -19.455566) -> (-68.699825, -20.06786)
  line L463 (-66.031357, -33.304241) -> (-65.686942, -34.135732)
  line L464 (-65.686942, -34.135732) -> (-68.273804, -35.207246)
  line L465 (-68.273804, -35.207246) -> (-68.962634, -33.544263)
  line L466 (-68.962634, -33.544263) -> (-66.375772, -32.472749)
  line L467 (-66.375772, -32.472749) -> (-66.031357, -33.304241)
  line L468 (-64.490308, -30.230535) -> (-63.0121, -29.618241)
  line L469 (-63.62927, -32.309264) -> (-64.490308, -30.230535)
  line L470 (-62.768232, -34.387993) -> (-63.62927, -32.309264)
  line L471 (-61.290025, -33.775699) -> (-62.768232, -34.387993)
  line L472 (-63.0121, -29.618241) -> (-61.290025, -33.775699)
  line L473 (-73.448423, -30.423333) -> (-72.491714, -32.733032)
  line L474 (-58.265599, -53.669405) -> (-59.39697, -54.800776)
  line L475 (-59.856589, -52.078414) -> (-58.265599, -53.669405)
  line L476 (-58.654507, -49.603541) -> (-57.381715, -50.876333)
  line L477 (-57.381715, -50.876333) -> (-55.401816, -48.896434)
  line L478 (-61.447579, -50.487424) -> (-59.856589, -52.078414)
  line L479 (-59.39697, -54.800776) -> (-62.57895, -51.618795)
  line L480 (-62.57895, -51.618795) -> (-61.447579, -50.487424)
  line L481 (-55.401816, -48.896434) -> (-56.038212, -48.260038)
  line L482 (-56.674609, -47.623642) -> (-58.654507, -49.603541)
  line L483 (-51.830927, -48.295393) -> (-57.982756, -54.447222)
  line L484 (-54.199735, -46.42156) -> (-52.608745, -48.01255)
  line L485 (-54.447222, -57.982756) -> (-48.295393, -51.830927)
  line L486 (-48.295393, -51.830927) -> (-51.830927, -48.295393)
  line L487 (-56.038212, -48.260038) -> (-56.674609, -47.623642)
  line L488 (-57.982756, -54.447222) -> (-56.214989, -56.214989)
  line L489 (-55.790725, -44.83057) -> (-54.199735, -46.42156)
  line L490 (-52.608745, -48.01255) -> (-51.477374, -46.88118)
  line L491 (-51.477374, -46.88118) -> (-54.659354, -43.699199)
  line L492 (-54.659354, -43.699199) -> (-55.790725, -44.83057)
  line L493 (-48.260038, -56.038212) -> (-47.623642, -56.674609)
  line L494 (-47.623642, -56.674609) -> (-49.603541, -58.654507)
  line L495 (-49.603541, -58.654507) -> (-50.876333, -57.381715)
  line L496 (-50.876333, -57.381715) -> (-48.896434, -55.401816)
  line L497 (-48.896434, -55.401816) -> (-48.260038, -56.038212)
  line L498 (-48.01255, -52.608745) -> (-46.88118, -51.477374)
  line L499 (-46.42156, -54.199735) -> (-48.01255, -52.608745)
  line L500 (-44.83057, -55.790725) -> (-46.42156, -54.199735)
  line L501 (-43.699199, -54.659354) -> (-44.83057, -55.790725)
  line L502 (-46.88118, -51.477374) -> (-43.699199, -54.659354)
  line L503 (-56.214989, -56.214989) -> (-54.447222, -57.982756)
  line L504 (-33.292002, -71.881344) -> (-33.904296, -73.359551)
  line L505 (-35.370731, -71.020306) -> (-33.292002, -71.881344)
  line L506 (-35.207246, -68.273804) -> (-33.544263, -68.962634)
  line L507 (-33.544263, -68.962634) -> (-32.472749, -66.375772)
  line L508 (-37.44946, -70.159268) -> (-35.370731, -71.020306)
  line L509 (-33.904296, -73.359551) -> (-38.061754, -71.637476)
  line L510 (-38.061754, -71.637476) -> (-37.44946, -70.159268)
  line L511 (-32.472749, -66.375772) -> (-33.304241, -66.031357)
  line L512 (-34.135732, -65.686942) -> (-35.207246, -68.273804)
  line L513 (-29.403686, -64.453962) -> (-32.733032, -72.491714)
  line L514 (-32.309264, -63.62927) -> (-30.230535, -64.490308)
  line L515 (-28.113634, -74.405131) -> (-24.784288, -66.367379)
  line L516 (-24.784288, -66.367379) -> (-29.403686, -64.453962)
  line L517 (-33.304241, -66.031357) -> (-34.135732, -65.686942)
  line L518 (-32.733032, -72.491714) -> (-30.423333, -73.448423)
  line L519 (-34.387993, -62.768232) -> (-32.309264, -63.62927)
  line L520 (-30.230535, -64.490308) -> (-29.618241, -63.0121)
  line L521 (-29.618241, -63.0121) -> (-33.775699, -61.290025)
  line L522 (-33.775699, -61.290025) -> (-34.387993, -62.768232)
  line L523 (-23.141566, -70.240874) -> (-22.310074, -70.585289)
  line L524 (-22.310074, -70.585289) -> (-23.381588, -73.172152)
  line L525 (-23.381588, -73.172152) -> (-25.044571, -72.483322)
  line L526 (-25.044571, -72.483322) -> (-23.973057, -69.896459)
  line L527 (-23.973057, -69.896459) -> (-23.141566, -70.240874)
  line L528 (-24.225318, -66.97775) -> (-23.613024, -65.499543)
  line L529 (-22.146589, -67.838788) -> (-24.225318, -66.97775)
  line L530 (-20.06786, -68.699825) -> (-22.146589, -67.838788)
  line L531 (-19.455566, -67.221618) -> (-20.06786, -68.699825)
  line L532 (-23.613024, -65.499543) -> (-19.455566, -67.221618)
  line L533 (-30.423333, -73.448423) -> (-28.113634, -74.405131)
  line L534 (0, -53.15) -> (0, -42.15) construction
  line L535 (0, -42.15) -> (4.375, -42.15) construction
  line L536 (0, -35.5) -> (2.5, -35.5)
  line L537 (2.5, -35.5) -> (2.5, -26.8)
  line L538 (-2.5, -26.8) -> (-2.5, -35.5)
  line L539 (-3.25, -27.15) -> (-3.25, -25.55)
  line L540 (-5.5, -27.15) -> (-3.25, -27.15)
  line L541 (-4.6, -29.75) -> (-5.5, -29.75)
  line L542 (-4.6, -32.55) -> (-4.6, -29.75)
  line L543 (-3.25, -25.55) -> (-7.75, -25.55)
  line L544 (-7.75, -25.55) -> (-7.75, -27.15)
  line L545 (-7.75, -27.15) -> (-5.5, -27.15)
  line L546 (-5.5, -29.75) -> (-6.4, -29.75)
  line L547 (-6.4, -29.75) -> (-6.4, -32.55)
  line L548 (-6.4, -32.55) -> (-4.6, -32.55)
  line L549 (2.5, -26.8) -> (-2.5, -26.8)
  line L550 (5.5, -29.75) -> (6.4, -29.75)
  line L551 (6.4, -29.75) -> (6.4, -32.55)
  line L552 (6.4, -32.55) -> (4.6, -32.55)
  line L553 (4.6, -32.55) -> (4.6, -29.75)
  line L554 (4.6, -29.75) -> (5.5, -29.75)
  line L555 (3.25, -27.15) -> (3.25, -25.55)
  line L556 (5.5, -27.15) -> (3.25, -27.15)
  line L557 (7.75, -27.15) -> (5.5, -27.15)
  line L558 (3.25, -25.55) -> (7.75, -25.55)
  line L559 (7.75, -25.55) -> (7.75, -27.15)
  line L560 (-2.5, -35.5) -> (0, -35.5)
  line L561 (-7.75, -35.15) -> (-5.5, -35.15)
  line L562 (-3.25, -36.75) -> (-7.75, -36.75)
  line L563 (-7.75, -36.75) -> (-7.75, -35.15)
  line L564 (-3.25, -35.15) -> (-3.25, -36.75)
  line L565 (0, -35.5) -> (0, -38.5) construction
  line L566 (-5.5, -35.15) -> (-3.25, -35.15)
  line L567 (0, -31.15) -> (0, -42.15) construction
  line L568 (57.15, -3.25) -> (58.75, -3.25)
  line L569 (58.75, -3.25) -> (58.75, -7.75)
  line L570 (57.15, -5.5) -> (57.15, -3.25)
  line L571 (57.15, -7.75) -> (57.15, -5.5)
  line L572 (58.75, -7.75) -> (57.15, -7.75)
  line L573 (54.55, -4.6) -> (54.55, -5.5)
  line L574 (54.55, -5.5) -> (54.55, -6.4)
  line L575 (51.75, -4.6) -> (54.55, -4.6)
  line L576 (51.75, -6.4) -> (51.75, -4.6)
  line L577 (54.55, -6.4) -> (51.75, -6.4)
  line L578 (49.15, -7.75) -> (49.15, -5.5)
  line L579 (49.15, -5.5) -> (49.15, -3.25)
  line L580 (47.55, -7.75) -> (49.15, -7.75)
  line L581 (47.55, -3.25) -> (47.55, -7.75)
  line L582 (49.15, -3.25) -> (47.55, -3.25)
  line L583 (48.8, -2.5) -> (48.8, 0)
  line L584 (48.8, 0) -> (45.8, 0) construction
  line L585 (53.15, 0) -> (42.15, 0) construction
  line L586 (48.8, 0) -> (48.8, 2.5)
  line L587 (48.8, 2.5) -> (57.5, 2.5)
  line L588 (57.5, -2.5) -> (48.8, -2.5)
  line L589 (57.5, 2.5) -> (57.5, -2.5)
  line L590 (54.55, 5.5) -> (54.55, 6.4)
  line L591 (54.55, 6.4) -> (51.75, 6.4)
  line L592 (51.75, 6.4) -> (51.75, 4.6)
  line L593 (58.75, 7.75) -> (57.15, 7.75)
  line L594 (51.75, 4.6) -> (54.55, 4.6)
  line L595 (54.55, 4.6) -> (54.55, 5.5)
  line L596 (57.15, 3.25) -> (58.75, 3.25)
  line L597 (57.15, 5.5) -> (57.15, 3.25)
  line L598 (58.75, 3.25) -> (58.75, 7.75)
  line L599 (57.15, 7.75) -> (57.15, 5.5)
  line L600 (27.15, -3.25) -> (25.55, -3.25)
  line L601 (26.8, 2.5) -> (26.8, -2.5)
  line L602 (27.15, 3.25) -> (25.55, 3.25)
  line L603 (32.55, 4.6) -> (29.75, 4.6)
  line L604 (29.75, 4.6) -> (29.75, 5.5)
  line L605 (27.15, 5.5) -> (27.15, 3.25)
  line L606 (29.75, 5.5) -> (29.75, 6.4)
  line L607 (25.55, 3.25) -> (25.55, 7.75)
  line L608 (25.55, 7.75) -> (27.15, 7.75)
  line L609 (27.15, 7.75) -> (27.15, 5.5)
  line L610 (29.75, 6.4) -> (32.55, 6.4)
  line L611 (32.55, 6.4) -> (32.55, 4.6)
  line L612 (27.15, -5.5) -> (27.15, -3.25)
  line L613 (35.5, 2.5) -> (26.8, 2.5)
  line L614 (35.5, 0) -> (35.5, 2.5)
  line L615 (25.55, -3.25) -> (25.55, -7.75)
  line L616 (25.55, -7.75) -> (27.15, -7.75)
  line L617 (27.15, -7.75) -> (27.15, -5.5)
  line L618 (26.8, -2.5) -> (35.5, -2.5)
  line L619 (29.75, -4.6) -> (29.75, -5.5)
  line L620 (32.55, -4.6) -> (29.75, -4.6)
  line L621 (29.75, -6.4) -> (32.55, -6.4)
  line L622 (32.55, -6.4) -> (32.55, -4.6)
  line L623 (35.15, -5.5) -> (35.15, -3.25)
  line L624 (35.15, -7.75) -> (35.15, -5.5)
  line L625 (36.75, -3.25) -> (36.75, -7.75)
  line L626 (36.75, -7.75) -> (35.15, -7.75)
  line L627 (29.75, -5.5) -> (29.75, -6.4)
  line L628 (42.15, 0) -> (42.15, 4.375) construction
  line L629 (35.15, -3.25) -> (36.75, -3.25)
  line L630 (35.5, 0) -> (38.5, 0) construction
  line L631 (35.5, -2.5) -> (35.5, 0)
  line L632 (31.15, 0) -> (42.15, 0) construction
  line L633 (3.25, 57.15) -> (3.25, 58.75)
  line L634 (3.25, 58.75) -> (7.75, 58.75)
  line L635 (5.5, 57.15) -> (3.25, 57.15)
  line L636 (7.75, 57.15) -> (5.5, 57.15)
  line L637 (7.75, 58.75) -> (7.75, 57.15)
  line L638 (4.6, 54.55) -> (5.5, 54.55)
  line L639 (5.5, 54.55) -> (6.4, 54.55)
  line L640 (4.6, 51.75) -> (4.6, 54.55)
  line L641 (6.4, 51.75) -> (4.6, 51.75)
  line L642 (6.4, 54.55) -> (6.4, 51.75)
  line L643 (7.75, 49.15) -> (5.5, 49.15)
  line L644 (5.5, 49.15) -> (3.25, 49.15)
  line L645 (7.75, 47.55) -> (7.75, 49.15)
  line L646 (3.25, 47.55) -> (7.75, 47.55)
  line L647 (3.25, 49.15) -> (3.25, 47.55)
  line L648 (2.5, 48.8) -> (0, 48.8)
  line L649 (0, 48.8) -> (0, 45.8) construction
  line L650 (0, 53.15) -> (0, 42.15) construction
  line L651 (0, 48.8) -> (-2.5, 48.8)
  line L652 (-2.5, 48.8) -> (-2.5, 57.5)
  line L653 (2.5, 57.5) -> (2.5, 48.8)
  line L654 (-2.5, 57.5) -> (2.5, 57.5)
  line L655 (-5.5, 54.55) -> (-6.4, 54.55)
  line L656 (-6.4, 54.55) -> (-6.4, 51.75)
  line L657 (-6.4, 51.75) -> (-4.6, 51.75)
  line L658 (-7.75, 58.75) -> (-7.75, 57.15)
  line L659 (-4.6, 51.75) -> (-4.6, 54.55)
  line L660 (-4.6, 54.55) -> (-5.5, 54.55)
  line L661 (-3.25, 57.15) -> (-3.25, 58.75)
  line L662 (-5.5, 57.15) -> (-3.25, 57.15)
  line L663 (-3.25, 58.75) -> (-7.75, 58.75)
  line L664 (-7.75, 57.15) -> (-5.5, 57.15)
  line L665 (3.25, 27.15) -> (3.25, 25.55)
  line L666 (-2.5, 26.8) -> (2.5, 26.8)
  line L667 (-3.25, 27.15) -> (-3.25, 25.55)
  line L668 (-4.6, 32.55) -> (-4.6, 29.75)
  line L669 (-4.6, 29.75) -> (-5.5, 29.75)
  line L670 (-5.5, 27.15) -> (-3.25, 27.15)
  line L671 (-5.5, 29.75) -> (-6.4, 29.75)
  line L672 (-3.25, 25.55) -> (-7.75, 25.55)
  line L673 (-7.75, 25.55) -> (-7.75, 27.15)
  line L674 (-7.75, 27.15) -> (-5.5, 27.15)
  line L675 (-6.4, 29.75) -> (-6.4, 32.55)
  line L676 (-6.4, 32.55) -> (-4.6, 32.55)
  line L677 (5.5, 27.15) -> (3.25, 27.15)
  line L678 (-2.5, 35.5) -> (-2.5, 26.8)
  line L679 (0, 35.5) -> (-2.5, 35.5)
  line L680 (3.25, 25.55) -> (7.75, 25.55)
  line L681 (7.75, 25.55) -> (7.75, 27.15)
  line L682 (7.75, 27.15) -> (5.5, 27.15)
  line L683 (2.5, 26.8) -> (2.5, 35.5)
  line L684 (4.6, 29.75) -> (5.5, 29.75)
  line L685 (4.6, 32.55) -> (4.6, 29.75)
  line L686 (6.4, 29.75) -> (6.4, 32.55)
  line L687 (6.4, 32.55) -> (4.6, 32.55)
  line L688 (5.5, 35.15) -> (3.25, 35.15)
  line L689 (7.75, 35.15) -> (5.5, 35.15)
  line L690 (3.25, 36.75) -> (7.75, 36.75)
  line L691 (7.75, 36.75) -> (7.75, 35.15)
  line L692 (5.5, 29.75) -> (6.4, 29.75)
  line L693 (0, 42.15) -> (-4.375, 42.15) construction
  line L694 (3.25, 35.15) -> (3.25, 36.75)
  line L695 (0, 35.5) -> (0, 38.5) construction
  line L696 (2.5, 35.5) -> (0, 35.5)
  line L697 (0, 31.15) -> (0, 42.15) construction
  line L698 (-57.15, 3.25) -> (-58.75, 3.25)
  line L699 (-58.75, 3.25) -> (-58.75, 7.75)
  line L700 (-57.15, 5.5) -> (-57.15, 3.25)
  line L701 (-57.15, 7.75) -> (-57.15, 5.5)
  line L702 (-58.75, 7.75) -> (-57.15, 7.75)
  line L703 (-54.55, 4.6) -> (-54.55, 5.5)
  line L704 (-54.55, 5.5) -> (-54.55, 6.4)
  line L705 (-51.75, 4.6) -> (-54.55, 4.6)
  line L706 (-51.75, 6.4) -> (-51.75, 4.6)
  line L707 (-54.55, 6.4) -> (-51.75, 6.4)
  line L708 (-49.15, 7.75) -> (-49.15, 5.5)
  line L709 (-49.15, 5.5) -> (-49.15, 3.25)
  line L710 (-47.55, 7.75) -> (-49.15, 7.75)
  line L711 (-47.55, 3.25) -> (-47.55, 7.75)
  line L712 (-49.15, 3.25) -> (-47.55, 3.25)
  line L713 (-48.8, 2.5) -> (-48.8, 0)
  line L714 (-48.8, 0) -> (-45.8, 0) construction
  line L715 (-53.15, 0) -> (-42.15, 0) construction
  line L716 (-48.8, 0) -> (-48.8, -2.5)
  line L717 (-48.8, -2.5) -> (-57.5, -2.5)
  line L718 (-57.5, 2.5) -> (-48.8, 2.5)
  line L719 (-57.5, -2.5) -> (-57.5, 2.5)
  line L720 (-54.55, -5.5) -> (-54.55, -6.4)
  line L721 (-54.55, -6.4) -> (-51.75, -6.4)
  line L722 (-51.75, -6.4) -> (-51.75, -4.6)
  line L723 (-58.75, -7.75) -> (-57.15, -7.75)
  line L724 (-51.75, -4.6) -> (-54.55, -4.6)
  line L725 (-54.55, -4.6) -> (-54.55, -5.5)
  line L726 (-57.15, -3.25) -> (-58.75, -3.25)
  line L727 (-57.15, -5.5) -> (-57.15, -3.25)
  line L728 (-58.75, -3.25) -> (-58.75, -7.75)
  line L729 (-57.15, -7.75) -> (-57.15, -5.5)
  line L730 (-27.15, 3.25) -> (-25.55, 3.25)
  line L731 (-26.8, -2.5) -> (-26.8, 2.5)
  line L732 (-27.15, -3.25) -> (-25.55, -3.25)
  line L733 (-32.55, -4.6) -> (-29.75, -4.6)
  line L734 (-29.75, -4.6) -> (-29.75, -5.5)
  line L735 (-27.15, -5.5) -> (-27.15, -3.25)
  line L736 (-29.75, -5.5) -> (-29.75, -6.4)
  line L737 (-25.55, -3.25) -> (-25.55, -7.75)
  line L738 (-25.55, -7.75) -> (-27.15, -7.75)
  line L739 (-27.15, -7.75) -> (-27.15, -5.5)
  line L740 (-29.75, -6.4) -> (-32.55, -6.4)
  line L741 (-32.55, -6.4) -> (-32.55, -4.6)
  line L742 (-27.15, 5.5) -> (-27.15, 3.25)
  line L743 (-35.5, -2.5) -> (-26.8, -2.5)
  line L744 (-35.5, 0) -> (-35.5, -2.5)
  line L745 (-25.55, 3.25) -> (-25.55, 7.75)
  line L746 (-25.55, 7.75) -> (-27.15, 7.75)
  line L747 (-27.15, 7.75) -> (-27.15, 5.5)
  line L748 (-26.8, 2.5) -> (-35.5, 2.5)
  line L749 (-29.75, 4.6) -> (-29.75, 5.5)
  line L750 (-32.55, 4.6) -> (-29.75, 4.6)
  line L751 (-29.75, 6.4) -> (-32.55, 6.4)
  line L752 (-32.55, 6.4) -> (-32.55, 4.6)
  line L753 (-35.15, 5.5) -> (-35.15, 3.25)
  line L754 (-35.15, 7.75) -> (-35.15, 5.5)
  line L755 (-36.75, 3.25) -> (-36.75, 7.75)
  line L756 (-36.75, 7.75) -> (-35.15, 7.75)
  line L757 (-29.75, 5.5) -> (-29.75, 6.4)
  line L758 (-42.15, 0) -> (-42.15, -4.375) construction
  line L759 (-35.15, 3.25) -> (-36.75, 3.25)
  line L760 (-35.5, 0) -> (-38.5, 0) construction
  line L761 (-35.5, 2.5) -> (-35.5, 0)
  line L762 (-31.15, 0) -> (-42.15, 0) construction
  point P0 (-5.5, -75.15)
  point P1 (5.5, -75.15)
  point P2 (-5.5, -79.95)
  point P3 (5.5, -70.35)
  point P4 (-5.5, -70.35)
  point P5 (21.840442, -67.099684)
  point P6 (32.003117, -62.890166)
  point P7 (25.514203, -75.968928)
  point P8 (33.839997, -67.324788)
  point P9 (23.677323, -71.534306)
  point P10 (28.75866, -69.429547)
  point P11 (45.855875, -53.634049)
  point P12 (53.634049, -45.855875)
  point P13 (52.6441, -60.422274)
  point P14 (57.028162, -49.249987)
  point P15 (49.249987, -57.028162)
  point P16 (53.139075, -53.139075)
  point P17 (62.890166, -32.003117)
  point P18 (67.099684, -21.840442)
  point P19 (71.75941, -35.676878)
  point P20 (71.534306, -23.677323)
  point P21 (67.324788, -33.839997)
  point P22 (69.429547, -28.75866)
  point P23 (21.840442, 0)
  point P24 (23.677323, 0)
  point P25 (25.514203, 0)
  point P26 (28.75866, 0)
  point P27 (32.003117, 0)
  point P28 (33.839997, 0)
  point P29 (45.855875, 0)
  point P30 (49.249987, 0)
  point P31 (52.6441, 0)
  point P32 (53.139075, 0)
  point P33 (53.634049, 0)
  point P34 (57.028162, 0)
  point P35 (62.890166, 0)
  point P36 (67.099684, 0)
  point P37 (69.429547, 0)
  point P38 (67.324788, 0)
  point P39 (71.534306, 0)
  point P40 (71.75941, 0)
  point P41 (0, 66.15)
  point P42 (-5.5, -53.15)
  point P43 (5.5, -53.15)
  point P44 (-5.5, -48.35)
  point P45 (5.5, -57.95)
  point P46 (-5.5, -57.95)
  point P47 (21.840442, -61.200316)
  point P48 (70.35, -5.5)
  point P49 (70.35, 5.5)
  point P50 (79.95, -5.5)
  point P51 (75.15, 5.5)
  point P52 (75.15, -5.5)
  point P53 (75.15, 0)
  point P54 (67.099684, 21.840442)
  point P55 (62.890166, 32.003117)
  point P56 (75.968928, 25.514203)
  point P57 (67.324788, 33.839997)
  point P58 (71.534306, 23.677323)
  point P59 (69.429547, 28.75866)